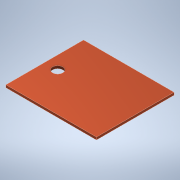
# Autodesk Inventor part: Tank resistive sensor
Saved by Autodesk Inventor 2022 (Build 260153000, 153)
## iProperties
Created: 2022-10-12
Part Number: Tank resistive sensor
Material: Ogólny
Document SubType Name: Modeling
Designer: kosak
Density: 1 g/cm^3
Appearance: Miedź — satynowa
Author: kosak
Autodesk Inventor part; units mm, degrees
ref_plane "YZ Plane" through (0, 0, 0) normal (1, 0, 0) x (0, 1, 0)
ref_plane "XZ Plane" through (0, 0, 0) normal (0, 1, 0) x (-1, 0, 0)
ref_plane "XY Plane" through (0, 0, 0) normal (0, 0, 1) x (1, 0, 0)
sketch "Szkic1" plane through (0, 0, 0) normal (0, 1, 0) x (-1, 0, 0)
  line L0 (0, 0) -> (35, 0)
  line L1 (35, 0) -> (35, -30)
  line L2 (35, -30) -> (0, -30)
  line L3 (0, -30) -> (0, 0)
  dimension "d0" = 35
  dimension "d1" = 30
  constraints: 8 end point, 2 parallel, 1 horizontal, 1 perpendicular
  measures "d0" distance of L1.end L2.end
  measures "d1" distance of L0.end L1.end
extrude "Wyciągnięcie proste1" add sketch "Szkic1" along normal blind 1
sketch "Szkic2" plane through (0, 1, 0) normal (0, 1, 0) x (1, 0, 0)
  line L0 (-35, 30) -> (-35, 0) projected
  line L1 (-35, 15) -> (-30, 15)
  circle A0 centre (-30, 15) radius 2
  point P0 (0, 0)
  dimension "d4" = 5
  dimension "d5" = 4
  constraints: 2 end point, 1 centre point, 1 coincident, 1 horizontal, 1 midpoint
  measures "d4" distance of L1.start L1.end
  measures "d5" diameter of A0
extrude "Wyciągnięcie proste2" cut sketch "Szkic2" against normal blind 1
